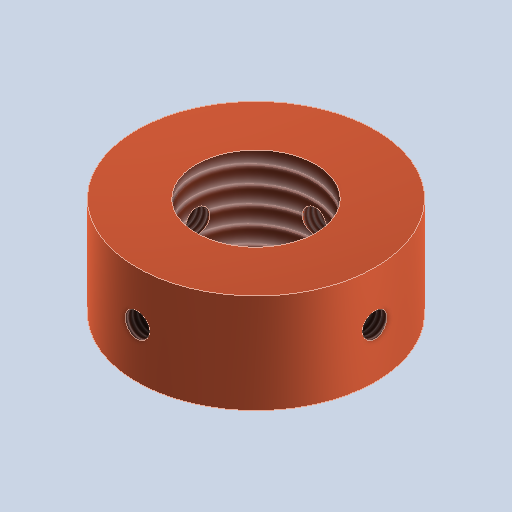
# Autodesk Inventor part: 36
Saved by Autodesk Inventor 2025.1 (Build 291241000, 241)
## iProperties
Created: 2024-09-17
Part Number: 36
Material: Copper
Document SubType Name: Modeling
Designer: ffogue
Density: 8.94 g/cm^3
Appearance: Copper - Satin
Author: ffogue
Autodesk Inventor part; units mm, degrees
ref_plane "XZ Plane" through (0, 0, 0) normal (0, 1, 0) x (-1, 0, 0)
ref_plane "XY Plane" through (0, 0, 0) normal (0, 0, 1) x (1, 0, 0)
sketch "Sketch1" plane through (0, 0, 0) normal (0, 0, 1) x (1, 0, 0)
  circle A0 centre (0, 0) radius 12
  circle A1 centre (0, 0) radius 6
  dimension "d0" = 24
  dimension "d1" = 12
  constraints: 2 centre point, 2 coincident
  measures "d0" diameter of A0
  measures "d1" diameter of A1
extrude "Extrusion1" add sketch "Sketch1" along normal mid plane 10
thread "Thread1" size "M12x1.75" class "6H" standard "ISO Metric profile" length 10
ref_plane "Work Plane1" through (12, 0, 0) normal (1, 0, 0) x (0, 1, 0)
sketch "Sketch2" plane through (12, 0, 0) normal (1, 0, 0) x (0, 1, 0)
  point P0 (0, 0)
  point P1 (0, 0)
  constraints: 1 coincident
hole "Hole1" at (12, 0, 0) direction (-1, 0, 0) diameter 2.459 depth 6.5 thread size "M3x0.5" class "6H" standard "ISO Metric profile"
pattern_circular "Circular Pattern1" count 4 over 360 about axis through (0, 0, 0) along (0, 0, 1) of "Hole1"
body "Solid1"
